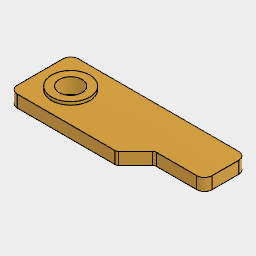
X_End_Stop_Flag_F01 (Autodesk Fusion 360 design; units mm, degrees)
Autodesk Fusion 360 part; units mm, degrees
sketch "スケッチ1" plane through (0, 0, 0) normal (0, 0, 1) x (1, 0, 0)
  line L0 (-4, -4) -> (10, -4)
  line L1 (10, -4) -> (12.5, -1.5)
  line L2 (12.5, -1.5) -> (19, -1.5)
  line L3 (19, -1.5) -> (19, 4)
  line L4 (19, 4) -> (-4, 4)
  line L5 (-4, 4) -> (-4, -4)
  line L6 (-4, 0) -> (0, 0) construction
  circle A0 centre (0, 0) radius 1.5
  circle A1 centre (0, 0) radius 2.5
  dimension "d1" = 23
  dimension "d2" = 8
  dimension "d3" = 5.5
  dimension "d4" = 14
  dimension "d5" = 45
  dimension "d6" = 4
  dimension "d7" = 3
  dimension "d8" = 5
  measures "d1" distance of L3.end L4.end
  measures "d2" distance of L0.start L4.end
  measures "d3" distance of L2.end L3.end
  measures "d4" distance of L0.start L0.end
  measures "d5" angle of L0 L1
  measures "d6" distance of L6.start L6.end
  measures "d7" diameter of A0
  measures "d8" diameter of A1
extrude "押し出し1" add sketch "スケッチ1" along normal blind 1.6 contours L0 L1 L2 L3 L4 L5
extrude "押し出し2" add sketch "スケッチ1" along normal blind 2 contours A1
fillet "フィレット1" radius 1 4 edges at (-4, 4, 0.8) (19, 4, 0.8) (19, -1.5, 0.8) (-4, -4, 0.8)
fillet "フィレット2" radius 0.5 2 edges at (12.5, -1.5, 0.8) (10, -4, 0.8)
